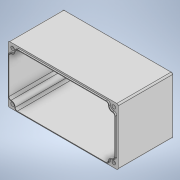
# Autodesk Inventor part: CustomBox_Rev3a
Saved by Autodesk Inventor 2021 (Build 250183000, 183)
## iProperties
Created: 2021-04-04
Part Number: CustomBox_Rev3a
Material: Generic
Document SubType Name: Modeling
Designer: James
Density: 1 g/cm^3
Appearance: Default
Author: James
Autodesk Inventor part; units mm, degrees
ref_plane "YZ Plane" through (0, 0, 0) normal (1, 0, 0) x (0, 1, 0)
ref_plane "XZ Plane" through (0, 0, 0) normal (0, 1, 0) x (-1, 0, 0)
ref_plane "XY Plane" through (0, 0, 0) normal (0, 0, 1) x (1, 0, 0)
sketch "Sketch2" plane through (0, 0, 0) normal (0, 0, 1) x (1, 0, 0)
  line L0 (-78, 40.5) -> (78, 40.5)
  line L1 (78, 40.5) -> (78, -40.5)
  line L2 (78, -40.5) -> (-78, -40.5)
  line L3 (-78, -40.5) -> (-78, 40.5)
  line L4 (-78, 40.5) -> (78, -40.5) construction
  line L5 (78, 40.5) -> (-78, -40.5) construction
  line L6 (0, 40.5) -> (0, -40.5)
  line L7 (-78, 0) -> (78, 0)
  circle A0 centre (-71.818, 34.318) radius 2.5
  line L8 (-75, 29.545) -> (-67.045, 29.545) construction
  line L9 (-67.045, 29.545) -> (-67.045, 37.5) construction
  line L10 (75, 37.5) -> (-63.0835, 37.5) construction
  line L11 (-75, 25.5835) -> (-75, -37.5) construction
  line L12 (-75, -37.5) -> (75, -37.5) construction
  line L13 (75, -37.5) -> (75, 37.5) construction
  line L14 (-75, 37.5) -> (-67.045, 29.545) construction
  arc A1 (-71.9375, 28.5829) -> (-66.0829, 34.4375) centre (-71.818, 34.318) ccw
  arc A2 (-71.9375, 28.5829) -> (-75, 25.5835) centre (-72, 25.5835) ccw
  arc A3 (-63.0835, 37.5) -> (-66.0829, 34.4375) centre (-63.0835, 34.5) ccw
  line L15 (-75, 25.5835) -> (-75, 0)
  line L16 (-63.0835, 37.5) -> (0, 37.5)
  arc A4 (-66.0829, -34.4375) -> (-71.9375, -28.5829) centre (-71.818, -34.318) ccw
  arc A5 (-75, -25.5835) -> (-71.9375, -28.5829) centre (-72, -25.5835) ccw
  arc A6 (-66.0829, -34.4375) -> (-63.0835, -37.5) centre (-63.0835, -34.5) ccw
  line L17 (-75, -25.5835) -> (-75, 0)
  line L18 (-63.0835, -37.5) -> (0, -37.5)
  arc A7 (66.0829, 34.4375) -> (71.9375, 28.5829) centre (71.818, 34.318) ccw
  arc A8 (75, 25.5835) -> (71.9375, 28.5829) centre (72, 25.5835) ccw
  arc A9 (66.0829, 34.4375) -> (63.0835, 37.5) centre (63.0835, 34.5) ccw
  line L19 (75, 25.5835) -> (75, 0)
  line L20 (63.0835, 37.5) -> (0, 37.5)
  line L21 (63.0835, -37.5) -> (0, -37.5)
  arc A10 (63.0835, -37.5) -> (66.0829, -34.4375) centre (63.0835, -34.5) ccw
  arc A11 (71.9375, -28.5829) -> (66.0829, -34.4375) centre (71.818, -34.318) ccw
  arc A12 (71.9375, -28.5829) -> (75, -25.5835) centre (72, -25.5835) ccw
  line L22 (75, -25.5835) -> (75, 0)
  circle A13 centre (-71.818, -34.318) radius 2.5
  circle A14 centre (71.818, 34.318) radius 2.5
  circle A15 centre (71.818, -34.318) radius 2.5
  line L23 (0, 37.5) -> (-75, 37.5) construction
  line L24 (-75, 0) -> (-75, 37.5) construction
  point P0 (0, 0)
  point P1 (-75, 29.545)
  dimension "d5" = 156
  dimension "d6" = 81
  dimension "d11" = 5
  dimension "d23" = 3
  dimension "lid_screw_offset_w" = 3.182
  dimension "d26" = 7.955
  dimension "d27" = 7.955
  dimension "d28" = 3
  constraints: 50 end point, 26 point on circle, 26 symmetric about line, 16 centre point, 10 point on line, 6 midpoint, 4 parallel, 4 perpendicular, 4 tangent, 3 horizontal, 1 coincident, 1 equal radius, 15 other
  measures "d5" distance of L1.end L2.end
  measures "d6" distance of L0.end L1.end
  measures "d11" diameter of A0
  measures "d23" distance between parallel lines of L0 L10
  measures "lid_screw_offset_w" distance from line of A0.centre L11
  measures "d26" distance between parallel lines of L9 L11
  measures "d27" distance between parallel lines of L8 L10
  measures "d28" radius of A2
extrude "Extrusion1" add sketch "Sketch2" against normal blind 3 contours L0 L6 L16 A3 A1 A2 L15 L7 L3 | L0 L1 L7 L19 A8 A7 A9 L20 L6 | L7 L17 A5 A4 A6 L18 L6 L2 L3 | L20 A9 A7 A8 L19 L7 L6 | L6 L7 L15 A2 A1 A3 L16 | L7 L6 L18 A6 A4 A5 L17 | L1 L2 L6 L21 A10 A11 A12 L22 L7 | L7 L22 A12 A11 A10 L21 L6 | A0 | A13 | A14 | A15
extrude "Extrusion2" add sketch "Sketch2" along normal blind 75 contours L0 L6 L16 A3 A1 A2 L15 L7 L3 | L0 L1 L7 L19 A8 A7 A9 L20 L6 | L7 L17 A5 A4 A6 L18 L6 L2 L3 | L1 L2 L6 L21 A10 A11 A12 L22 L7
fillet "Fillet1" radius 2 4 edges at (-78, 40.5, 36) (-78, -40.5, 36) (78, -40.5, 36) (78, 40.5, 36)
fillet "Fillet2" radius 1 16 edges at (-65.2268, 36.5991, 0) (-67.7618, 30.2618, 0) (-74.0991, 27.7268, 0) (-75, 0, 0) (-74.0991, -27.7268, 0) (-67.7618, -30.2618, 0) (-65.2268, -36.5991, 0) (0, -37.5, 0) (65.2268, -36.5991, 0) (67.7618, -30.2618, 0) (74.0991, -27.7268, 0) (75, 0, 0) (74.0991, 27.7268, 0) (67.7618, 30.2618, 0) (65.2268, 36.5991, 0) (0, 37.5, 0)
fillet "Fillet3" radius 1 8 edges at (-77.4142, 39.9142, -3) (0, 40.5, -3) (77.4142, 39.9142, -3) (78, 0, -3) (77.4142, -39.9142, -3) (0, -40.5, -3) (-77.4142, -39.9142, -3) (-78, 0, -3)
ref_plane "Work Plane1" through (78, -40.5, 0) normal (0, 0, -1) x (-1, 0, 0)
sketch "Sketch3" plane through (78, -40.5, 0) normal (0, 0, -1) x (-1, 0, 0)
  line L0 (156, 79) -> (156, 2) projected
  line L1 (154, 0) -> (2, 0) projected
  line L2 (2, 81) -> (154, 81) projected
  line L3 (0, 2) -> (0, 79) projected
  line L4 (78, 81) -> (78, 0) projected
  line L5 (156, 40.5) -> (0, 40.5) projected
  line L6 (14.9165, 4) -> (141.0835, 4) projected
  line L7 (152, 14.9165) -> (152, 66.0835) projected
  line L8 (141.0835, 77) -> (14.9165, 77) projected
  line L9 (4, 66.0835) -> (4, 14.9165) projected
  arc A0 (12.9169, 6.0417) -> (6.0417, 12.9169) centre (6.182, 6.182) ccw projected
  arc A1 (6.0417, 68.0831) -> (12.9169, 74.9583) centre (6.182, 74.818) ccw projected
  arc A2 (143.0831, 74.9583) -> (149.9583, 68.0831) centre (149.818, 74.818) ccw projected
  arc A3 (149.9583, 12.9169) -> (143.0831, 6.0417) centre (149.818, 6.182) ccw projected
  circle A4 centre (136.0835, 9) radius 1.25
  circle A5 centre (136.0835, 9) radius 2.25
  circle A6 centre (136.0835, 72) radius 1.25
  circle A7 centre (136.0835, 72) radius 2.25
  circle A8 centre (19.9165, 9) radius 1.25
  circle A9 centre (19.9165, 9) radius 2.25
  circle A10 centre (19.9165, 72) radius 1.25
  circle A11 centre (19.9165, 72) radius 2.25
  circle A12 centre (147, 40.5) radius 1.25
  circle A13 centre (147, 40.5) radius 2.25
  circle A14 centre (9, 40.5) radius 1.25
  circle A15 centre (9, 40.5) radius 2.25
  circle A16 centre (78, 9) radius 1.25
  circle A17 centre (78, 9) radius 2.25
  circle A18 centre (78, 72) radius 1.25
  circle A19 centre (78, 72) radius 2.25
  point P0 (78, 40.5)
  point P1 (14.9165, 6)
  point P2 (6, 14.9165)
  point P3 (6, 66.0835)
  point P4 (14.9165, 75)
  point P5 (141.0835, 75)
  point P6 (150, 66.0835)
  point P7 (150, 14.9165)
  point P8 (141.0835, 6)
  dimension "mounting_hole_d" = 2.5
  dimension "d37" = 4.5
  dimension "d38" = 5
  dimension "d39" = 5
  dimension "d40" = 2.5
  dimension "d41" = 4.5
  dimension "mounting_hole_offset" = 5
  dimension "d43" = 2.5
  dimension "d44" = 4.5
  dimension "d45" = 5
  constraints: 16 centre point, 10 symmetric about line, 8 coincident, 2 point on line, 10 other
  measures "mounting_hole_d" diameter of A4
  measures "d37" diameter of A5
  measures "d38" distance from line of L6 A4.centre
  measures "d39" horizontal distance of L6.end A4.centre
  measures "d40" diameter of A12
  measures "d41" diameter of A13
  measures "mounting_hole_offset" distance from line of L7 A12.centre
  measures "d43" diameter of A16
  measures "d44" diameter of A17
  measures "d45" distance from line of L6 A16.centre
extrude "Extrusion3" add sketch "Sketch3" against normal blind 4 contours A19 L4 A18 | L4 A18 A19 | A18 L4 | L4 A18 | A17 L4 A16 | L4 A16 A17 | A16 L4 | L4 A16 | A13 L5 A12 | L5 A12 A13 | A12 L5 | L5 A12 | A15 L5 A14 | L5 A14 A15 | A14 L5 | L5 A14 | A4 | A5 | A6 | A7 | A8 | A9 | A10 | A11
extrude "Extrusion4" cut sketch "Sketch3" against normal blind 4 contours A18 L4 | L4 A18 | A16 L4 | L4 A16 | A12 L5 | L5 A12 | A14 L5 | L5 A14 | A4 | A6 | A8 | A10
fillet "Fillet4" radius 1.5 8 edges at (-55.8335, -31.5, 0) (-66.75, 0, 0) (2.25, -31.5, 0) (60.3335, -31.5, 0) (-55.8335, 31.5, 0) (2.25, 31.5, 0) (60.3335, 31.5, 0) (71.25, 0, 0)
sketch "Sketch4" plane through (0, 0, 75) normal (0, 0, 1) x (1, 0, 0)
  line L0 (75, 25.5835) -> (75, -25.5835) projected
  arc A0 (71.9375, -28.5829) -> (75, -25.5835) centre (72, -25.5835) ccw projected
  arc A1 (71.9375, -28.5829) -> (66.0829, -34.4375) centre (71.818, -34.318) ccw projected
  arc A2 (63.0835, -37.5) -> (66.0829, -34.4375) centre (63.0835, -34.5) ccw projected
  line L1 (63.0835, -37.5) -> (-63.0835, -37.5) projected
  arc A3 (-66.0829, -34.4375) -> (-63.0835, -37.5) centre (-63.0835, -34.5) ccw projected
  arc A4 (-66.0829, -34.4375) -> (-71.9375, -28.5829) centre (-71.818, -34.318) ccw projected
  arc A5 (-75, -25.5835) -> (-71.9375, -28.5829) centre (-72, -25.5835) ccw projected
  line L2 (-75, -25.5835) -> (-75, 25.5835) projected
  arc A6 (-71.9375, 28.5829) -> (-75, 25.5835) centre (-72, 25.5835) ccw projected
  arc A7 (-71.9375, 28.5829) -> (-66.0829, 34.4375) centre (-71.818, 34.318) ccw projected
  arc A8 (-63.0835, 37.5) -> (-66.0829, 34.4375) centre (-63.0835, 34.5) ccw projected
  line L3 (-63.0835, 37.5) -> (63.0835, 37.5) projected
  arc A9 (66.0829, 34.4375) -> (63.0835, 37.5) centre (63.0835, 34.5) ccw projected
  arc A10 (66.0829, 34.4375) -> (71.9375, 28.5829) centre (71.818, 34.318) ccw projected
  arc A11 (75, 25.5835) -> (71.9375, 28.5829) centre (72, 25.5835) ccw projected
  line L4 (63.0835, 38.3) -> (-63.0835, 38.3)
  arc A12 (-63.0835, 38.3) -> (-66.8827, 34.4208) centre (-63.0835, 34.5) ccw
  arc A13 (-71.9208, 29.3827) -> (-66.8827, 34.4208) centre (-71.818, 34.318) ccw
  arc A14 (-71.9208, 29.3827) -> (-75.8, 25.5835) centre (-72, 25.5835) ccw
  line L5 (-75.8, 25.5835) -> (-75.8, -25.5835)
  arc A15 (-75.8, -25.5835) -> (-71.9208, -29.3827) centre (-72, -25.5835) ccw
  arc A16 (-66.8827, -34.4208) -> (-71.9208, -29.3827) centre (-71.818, -34.318) ccw
  arc A17 (-66.8827, -34.4208) -> (-63.0835, -38.3) centre (-63.0835, -34.5) ccw
  line L6 (-63.0835, -38.3) -> (63.0835, -38.3)
  arc A18 (63.0835, -38.3) -> (66.8827, -34.4208) centre (63.0835, -34.5) ccw
  arc A19 (71.9208, -29.3827) -> (66.8827, -34.4208) centre (71.818, -34.318) ccw
  arc A20 (71.9208, -29.3827) -> (75.8, -25.5835) centre (72, -25.5835) ccw
  line L7 (75.8, -25.5835) -> (75.8, 25.5835)
  arc A21 (75.8, 25.5835) -> (71.9208, 29.3827) centre (72, 25.5835) ccw
  arc A22 (66.8827, 34.4208) -> (71.9208, 29.3827) centre (71.818, 34.318) ccw
  arc A23 (66.8827, 34.4208) -> (63.0835, 38.3) centre (63.0835, 34.5) ccw
  point P0 (0, 0)
  dimension "inner_gasket_wall" = 0.8
  constraints: 24 point on circle, 12 centre point, 8 end point, 15 other
  measures "inner_gasket_wall" distance between parallel lines of L3 L4
extrude "Extrusion5" add sketch "Sketch4" along normal blind 2
equation "\"d5\" = box_length_outer"
equation "\"d6\" = box_width_outer"
equation "\"d23\" = wall_thickness"
equation "\"box_height\" = 75"
equation "\"wall_thickness\" = 3"
equation "\"box_length_outer\" = box_length + 2 * wall_thickness"
equation "\"box_width_outer\" = box_height + 2 * wall_thickness"
equation "\"lid_screw_d\" = 4"
equation "\"min_wall_width\" = 1"
equation "\"box_length\" = 150"
body "Solid1"
